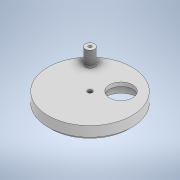
# Autodesk Inventor part: TopReactor
Saved by Autodesk Inventor 2022 (Build 260153070, 153G)
## iProperties
Created: 2021-07-20
Part Number: TopReactor
Material: Generic
Document SubType Name: Modeling
Designer: Eakawit_kor
Density: 1 g/cm^3
Appearance: Default
Author: Eakawit_kor
Autodesk Inventor part; units mm, degrees
ref_plane "YZ Plane" through (0, 0, 0) normal (1, 0, 0) x (0, 1, 0)
ref_plane "XZ Plane" through (0, 0, 0) normal (0, 1, 0) x (-1, 0, 0)
ref_plane "XY Plane" through (0, 0, 0) normal (0, 0, 1) x (1, 0, 0)
sketch "Sketch1" plane through (0, 0, 0) normal (0, 1, 0) x (-1, 0, 0)
  circle A0 centre (0, 0) radius 25
  dimension "d0" = 50
  constraints: 1 centre point, 1 coincident
  measures "d0" diameter of A0
extrude "Extrusion1" add sketch "Sketch1" along normal blind 2
sketch "Sketch3" plane through (0, 2, 0) normal (0, 1, 0) x (1, 0, 0)
  circle A0 centre (0, 0) radius 27
  circle A1 centre (0, 0) radius 25 projected
  dimension "d3" = 2
  constraints: 1 centre point, 1 coincident
  measures "d3" radial gap between concentric circles of A0 A1
extrude "Extrusion2" add sketch "Sketch3" along normal blind 6.5 contours A0 | A1
sketch "Sketch4" plane through (0, 8.5, 0) normal (0, 1, 0) x (1, 0, 0)
  circle A0 centre (0, 0) radius 1.5
  circle A1 centre (-15, 15) radius 1
  dimension "d6" = 3
  dimension "d8" = 15
  dimension "d9" = 15
  dimension "d10" = 2
  constraints: 2 centre point, 1 coincident
  measures "d6" diameter of A0
  measures "d8" horizontal distance of point (0, 0) A1.centre
  measures "d9" horizontal distance of point (0, 0) A1.centre
  measures "d10" diameter of A1
extrude "Extrusion3" cut sketch "Sketch4" against normal through all
sketch "Sketch5" plane through (0, 8.5, 0) normal (0, 1, 0) x (1, 0, 0)
  circle A0 centre (-15, 15) radius 3
  circle A1 centre (-15, 15) radius 1 projected
  point P0 (0, 0)
  dimension "d14" = 2
  constraints: 1 centre point, 1 concentric
  measures "d14" radial gap between concentric circles of A1 A0
extrude "Extrusion4" add sketch "Sketch5" along normal blind 10
thread "Thread1" size "M6x1" class "6g" standard "ANSI Metric M Profile" length 9
sketch "Sketch7" plane through (0, 8.5, 0) normal (0, 1, 0) x (1, 0, 0)
  circle A0 centre (10, 10) radius 10.55
  point P0 (0, 0)
  dimension "d21" = 21.1
  dimension "d22" = 10
  dimension "d23" = 10
  constraints: 1 centre point
  measures "d21" diameter of A0
  measures "d22" horizontal distance of A0.centre point (0, 0)
  measures "d23" horizontal distance of point (0, 0) A0.centre
extrude "Extrusion5" cut sketch "Sketch7" against normal through all
sketch "Sketch8" plane through (0, 8.5, 0) normal (0, 1, 0) x (1, 0, 0)
  circle A0 centre (10, 10) radius 10.55
  circle A1 centre (10, 10) radius 10.55 projected
  point P0 (0, 0)
  constraints: 2 concentric, 1 centre point
extrude "Extrusion6" add sketch "Sketch8" against normal blind 2.5
sketch "Sketch9" plane through (10, 6, -10) normal (0, -1, 0) x (1, 0, 0)
  circle A0 centre (0, 0) radius 7.4
  circle A1 centre (0, 0) radius 10.55 projected
  point P0 (-10, 10)
  dimension "d28" = 14.8
  constraints: 1 centre point, 1 concentric
  measures "d28" diameter of A0
extrude "Extrusion7" cut sketch "Sketch9" against normal up to surface (2.5 mm away) contours A0
body "Solid1"
